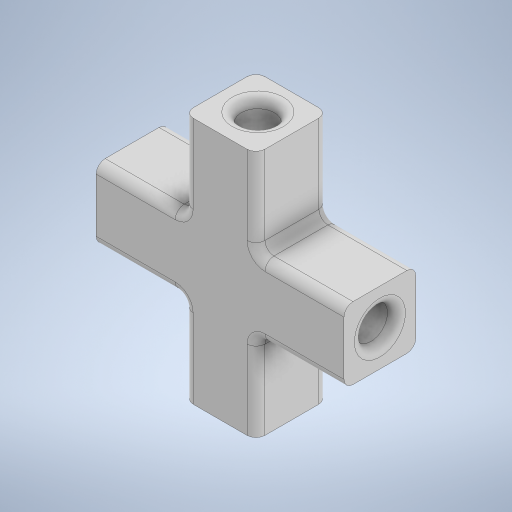
# Autodesk Inventor part: universal bağlantı
Saved by Autodesk Inventor 2023.2 (Build 272271000, 271)
## iProperties
Created: 2022-11-25
Part Number: universal bağlantı
Material: Generic
Document SubType Name: Modeling
Designer: omrfrkmll
Density: 1 g/cm^3
Appearance: Default
Author: omrfrkmll
Autodesk Inventor part; units mm, degrees
ref_plane "YZ Plane" through (0, 0, 0) normal (1, 0, 0) x (0, 1, 0)
ref_plane "XZ Plane" through (0, 0, 0) normal (0, 1, 0) x (-1, 0, 0)
ref_plane "XY Plane" through (0, 0, 0) normal (0, 0, 1) x (1, 0, 0)
sketch "Sketch1" plane through (0, 0, 0) normal (0, 0, 1) x (1, 0, 0)
  line L0 (-6.9, 6.9) -> (6.9, 6.9)
  line L1 (6.9, 6.9) -> (6.9, -6.9)
  line L2 (6.9, -6.9) -> (-6.9, -6.9)
  line L3 (-6.9, -6.9) -> (-6.9, 6.9)
  line L4 (0, 10.0373) -> (0, -9.8316)
  line L5 (-8.1862, 0) -> (13.9453, 0)
  line L6 (-6.9, 6.9) -> (-2, 6.9)
  line L7 (-2, 6.9) -> (-2, 2)
  line L8 (-2, 2) -> (-6.9, 2)
  line L9 (-6.9, 2) -> (-6.9, 6.9)
  line L10 (8.1862, 0) -> (-13.9453, 0)
  line L11 (2, 6.9) -> (2, 2)
  line L12 (2, 2) -> (6.9, 2)
  line L13 (0, -10.0373) -> (0, 9.8316)
  line L14 (-2, -6.9) -> (-2, -2)
  line L15 (-2, -2) -> (-6.9, -2)
  line L16 (2, -6.9) -> (2, -2)
  line L17 (2, -2) -> (6.9, -2)
  point P0 (0, 0)
  point P1 (-6.9, 2)
  point P2 (-6.9, -2)
  point P3 (-2, -6.9)
  point P4 (2, -6.9)
  point P5 (6.9, -2)
  point P6 (6.9, 2)
  point P7 (2, 6.9)
  dimension "d0" = 13.8
  dimension "d1" = 13.8
  dimension "d2" = 4
  dimension "d3" = 4
  constraints: 36 end point, 13 symmetric about line, 4 horizontal, 4 parallel, 2 perpendicular, 2 vertical, 3 other
  measures "d0" distance between parallel lines of L1 L3
  measures "d1" distance between parallel lines of L2 L0
  measures "d2" distance between parallel lines of L11 L7
  measures "d3" distance between parallel lines of L17 L12
extrude "Extrusion1" add sketch "Sketch1" along normal blind 4 contours L0 L4 L5 L3 L8 L7 | L0 L11 L12 L1 L5 L4 | L5 L4 L2 L14 L15 L3 | L5 L1 L17 L16 L2 L4
sketch "Sketch2" plane through (6.9, -2, 0) normal (1, 0, 0) x (0, 0, -1)
  circle A0 centre (-2, 2) radius 0.925
  line L0 (0, 0) -> (0, 4) projected
  line L1 (0, 4) -> (-4, 4) projected
  line L2 (-2, 4) -> (-2, 0)
  line L3 (0, 2) -> (-4.0632, 2)
  dimension "d6" = 1.85
  constraints: 4 end point, 2 midpoint, 1 centre point, 1 horizontal, 1 perpendicular, 1 point on line
  measures "d6" diameter of A0
extrude "Extrusion2" cut sketch "Sketch2" against normal up to surface (13.8 mm away) contours L3 L2 A0 | A0 L2 L3 | L2 L3 A0 | A0 L3 L2
sketch "Sketch3" plane through (-2, 6.9, 0) normal (0, 1, 0) x (1, 0, 0)
  line L0 (0, 0) -> (0, -4) projected
  line L1 (0, -1.8969) -> (5.1467, -1.8969)
  line L2 (0, -4) -> (4, -4) projected
  line L3 (2, -4) -> (2, 0.7903)
  circle A0 centre (2, -1.8969) radius 0.925
  point P0 (2, 0)
  dimension "d10" = 1.85
  constraints: 4 end point, 3 point on line, 2 horizontal, 2 vertical, 1 centre point, 1 midpoint
  measures "d10" diameter of A0
extrude "Extrusion3" cut sketch "Sketch3" against normal up to surface (13.8 mm away) contours A0 L3 L1 | L1 L3 A0 | L3 A0 L1 | L1 A0 L3
fillet "Fillet1" radius 0.5 8 edges at (-0.925, 6.9, 1.8969) (6.9, 0, 2.925) (-0.925, -6.9, 1.8969) (-6.9, 0, 2.925) (0.7098, -0.609, 1.3038) (-0.6115, -0.7116, 2.5909) (-0.6112, 0.7114, 2.5912) (0.7098, 0.609, 1.3038)
fillet "Fillet2" radius 0.5 20 edges at (2, -4.45, 4) (4.45, -2, 4) (2, -4.45, 0) (4.45, -2, 0) (2, -2, 2) (-2, -4.45, 4) (-2, -4.45, 0) (-2, -2, 2) (-4.45, -2, 4) (-4.45, -2, 0) (-4.45, 2, 4) (-2, 4.45, 4) (-2, 2, 2) (4.45, 2, 4) (2, 4.45, 4) (-2, 4.45, 0) (-4.45, 2, 0) (4.45, 2, 0) (2, 4.45, 0) (2, 2, 2)
body "Solid1"
